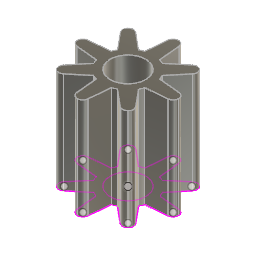
Small Body Gear (Autodesk Fusion 360 design; units mm, degrees)
Autodesk Fusion 360 part; units mm, degrees
note: some values were not read from the file. Set by a fixed rule: which sketch regions a step uses.
sketch "Small Body Gear" plane through (0, 0, 0) normal (0, 0, 1) x (1, 0, 0)
  circle A0 centre (0, 0) radius 0.875
  arc A1 (-0.583, -1.1057) -> (-0.3759, -1.1921) centre (0, 0) ccw
  arc A2 (-1.1941, -0.3696) -> (-1.1057, -0.583) centre (0, 0) ccw
  arc A3 (-1.1057, 0.583) -> (-1.1941, 0.3696) centre (0, 0) ccw
  arc A4 (-0.3696, 1.1941) -> (-0.583, 1.1057) centre (0, 0) ccw
  arc A5 (0.583, 1.1057) -> (0.3696, 1.1941) centre (0, 0) ccw
  arc A6 (1.1941, 0.3696) -> (1.1057, 0.583) centre (0, 0) ccw
  arc A7 (0.3696, -1.1941) -> (0.583, -1.1057) centre (0, 0) ccw
  arc A8 (1.1057, -0.583) -> (1.1941, -0.3696) centre (0, 0) ccw
  line L0 (1.767, -1.7685) -> (1.7678, -1.7678)
  line L1 (1.767, -1.7685) -> (1.7664, -1.7691)
  line L2 (2.5, 0) -> (2.5, 0.001)
  line L3 (2.5, 0) -> (2.5, -0.001)
  line L4 (1.7685, 1.767) -> (1.7678, 1.7678)
  line L5 (1.7685, 1.767) -> (1.7691, 1.7664)
  line L6 (0, 2.5) -> (-0.001, 2.5)
  line L7 (0, 2.5) -> (0.001, 2.5)
  line L8 (-1.767, 1.7685) -> (-1.7678, 1.7678)
  line L9 (-1.767, 1.7685) -> (-1.7664, 1.7691)
  line L10 (-2.5, 0) -> (-2.5, -0.001)
  line L11 (-2.5, 0) -> (-2.5, 0.001)
  line L12 (-1.7685, -1.767) -> (-1.7678, -1.7678)
  line L13 (-1.7685, -1.767) -> (-1.7691, -1.7664)
  line L14 (0, -2.5) -> (-0.001, -2.5)
  line L15 (0, -2.5) -> (-0.0002, -2.5)
  line L16 (-0.2739, -2.2513) -> (-0.3759, -1.1921)
  line L17 (0.2729, -2.2501) -> (0.3696, -1.1941)
  arc A9 (-0.2739, -2.2513) -> (-0.0002, -2.5) centre (-0.0002, -2.225) ccw
  arc A10 (-0.001, -2.5) -> (0.2729, -2.2501) centre (-0.001, -2.225) ccw
  line L18 (1.3973, -1.7845) -> (0.583, -1.1057)
  line L19 (1.7835, -1.3989) -> (1.1057, -0.583)
  arc A11 (1.3973, -1.7845) -> (1.7678, -1.7678) centre (1.5734, -1.5732) ccw
  arc A12 (1.7664, -1.7691) -> (1.7835, -1.3989) centre (1.572, -1.5746) ccw
  line L20 (1.1941, -0.3696) -> (2.2501, -0.2729)
  line L21 (2.2501, 0.2729) -> (1.1941, 0.3696)
  arc A13 (2.2501, -0.2729) -> (2.5, 0.001) centre (2.225, 0.001) ccw
  arc A14 (2.5, -0.001) -> (2.2501, 0.2729) centre (2.225, -0.001) ccw
  line L22 (1.1057, 0.583) -> (1.7845, 1.3973)
  line L23 (0.583, 1.1057) -> (1.3989, 1.7835)
  line L24 (0.3696, 1.1941) -> (0.2729, 2.2501)
  line L25 (-0.3696, 1.1941) -> (-0.2729, 2.2501)
  line L26 (-0.583, 1.1057) -> (-1.3973, 1.7845)
  line L27 (-1.1057, 0.583) -> (-1.7835, 1.3989)
  arc A15 (1.7845, 1.3973) -> (1.7678, 1.7678) centre (1.5732, 1.5734) ccw
  arc A16 (1.7691, 1.7664) -> (1.3989, 1.7835) centre (1.5746, 1.572) ccw
  arc A17 (0.2729, 2.2501) -> (-0.001, 2.5) centre (-0.001, 2.225) ccw
  arc A18 (0.001, 2.5) -> (-0.2729, 2.2501) centre (0.001, 2.225) ccw
  arc A19 (-1.3973, 1.7845) -> (-1.7678, 1.7678) centre (-1.5734, 1.5732) ccw
  arc A20 (-1.7664, 1.7691) -> (-1.7835, 1.3989) centre (-1.572, 1.5746) ccw
  line L28 (-1.1941, 0.3696) -> (-2.2501, 0.2729)
  line L29 (-1.1941, -0.3696) -> (-2.2501, -0.2729)
  line L30 (-1.1057, -0.583) -> (-1.7845, -1.3973)
  line L31 (-0.583, -1.1057) -> (-1.3989, -1.7835)
  arc A21 (-2.2501, 0.2729) -> (-2.5, -0.001) centre (-2.225, -0.001) ccw
  arc A22 (-2.5, 0.001) -> (-2.2501, -0.2729) centre (-2.225, 0.001) ccw
  arc A23 (-1.7691, -1.7664) -> (-1.3989, -1.7835) centre (-1.5746, -1.572) ccw
  arc A24 (-1.7845, -1.3973) -> (-1.7678, -1.7678) centre (-1.5732, -1.5734) ccw
  constraint coincident A0.centre A1.centre
  constraint concentric A0 A7
  constraint concentric A1 A7
  constraint concentric A2 A7
  constraint concentric A3 A7
  constraint concentric A4 A7
  constraint concentric A5 A7
  constraint concentric A6 A7
  constraint concentric A7 A8
  constraint parallel L14 L15
  constraint tangent L15 A9
  constraint tangent L16 A9
  constraint tangent L14 A10
  constraint tangent L17 A10
  constraint tangent L18 A11
  constraint tangent L0 A11
  constraint tangent L1 A12
  constraint tangent L19 A12
  constraint tangent L20 A13
  constraint tangent L2 A13
  constraint tangent L3 A14
  constraint tangent L21 A14
  constraint tangent L4 A15
  constraint tangent L22 A15
  constraint tangent L5 A16
  constraint tangent L23 A16
  constraint tangent L6 A17
  constraint tangent L24 A17
  constraint tangent L25 A18
  constraint tangent L7 A18
  constraint tangent L8 A19
  constraint tangent L26 A19
  constraint tangent L9 A20
  constraint tangent L27 A20
  constraint tangent L10 A21
  constraint tangent L28 A21
  constraint tangent L29 A22
  constraint tangent L11 A22
  constraint tangent L13 A23
  constraint tangent L31 A23
  constraint tangent L12 A24
  constraint tangent L30 A24
extrude "Extrude1" add sketch "Small Body Gear" along normal blind 5
named bodies: "Small Body Gear"
